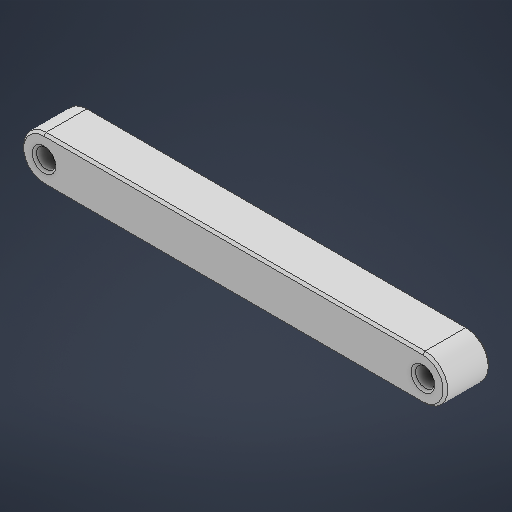
# Autodesk Inventor part: HeightAdjustment
Saved by Autodesk Inventor 2026.3 (Build 303398000, 398)
## iProperties
Created: 2026-06-24
Part Number: HeightAdjustment
Material: Generic
Document SubType Name: Modeling
Designer: frede
Density: 1 g/cm^3
Appearance: Default
Author: frede
Autodesk Inventor part; units mm, degrees
ref_plane "YZ Plane" through (0, 0, 0) normal (1, 0, 0) x (0, 1, 0)
ref_plane "XZ Plane" through (0, 0, 0) normal (0, 1, 0) x (-1, 0, 0)
ref_plane "XY Plane" through (0, 0, 0) normal (0, 0, 1) x (1, 0, 0)
sketch "Sketch1" plane through (0, 0, 0) normal (0, 0, 1) x (1, 0, 0)
  circle A0 centre (0, 0) radius 2.125
  circle A1 centre (84, 0) radius 2.125
  arc A2 (84, -5) -> (84, 5) centre (84, 0) ccw
  arc A3 (0, 5) -> (0, -5) centre (0, 0) ccw
  line L0 (0, 5) -> (84, 5)
  line L1 (0, -5) -> (84, -5)
  dimension "d0" = 4.25
  dimension "d1" = 4.25
  dimension "d2" = 10
  dimension "d3" = 10
  constraints: 4 centre point, 4 end point, 4 point on circle, 4 tangent, 3 coincident
  measures "d0" diameter of A0
  measures "d1" diameter of A1
  measures "d2" diameter of A2
  measures "d3" diameter of A3
extrude "Extrusion1" add sketch "Sketch1" along normal blind 10
chamfer "Chamfer1" distance 0.5 angle 45 12 edges at (-2.125, 0, 10) (-2.125, 0, 0) (42, -5, 0) (89, 0, 0) (42, 5, 0) (-5, 0, 0) (42, -5, 10) (89, 0, 10) (42, 5, 10) (-5, 0, 10) (81.875, 0, 10) (81.875, 0, 0)
body "Solid1"
